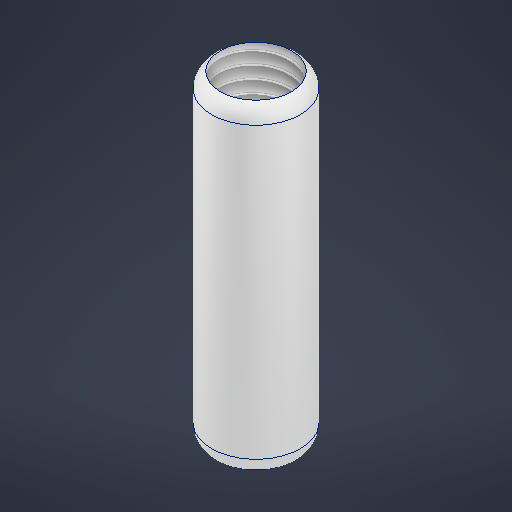
# Autodesk Inventor part: P_Gewindebuchse_M4_20
Saved by Autodesk Inventor 2026 (Build 300175000, 175)
## iProperties
Created: 2025-04-26
Part Number: P_Gewindebuchse_M4_20
Material: Aluminium 6061
Document SubType Name: Modeling
Designer: FAL
Density: 2.7 g/cm^3
Appearance: Aluminium - flach
Author: FAL
Autodesk Inventor part; units mm, degrees
ref_plane "YZ Plane" through (0, 0, 0) normal (1, 0, 0) x (0, 1, 0)
ref_plane "XZ Plane" through (0, 0, 0) normal (0, 1, 0) x (-1, 0, 0)
ref_plane "XY Plane" through (0, 0, 0) normal (0, 0, 1) x (1, 0, 0)
sketch "Skizze1" plane through (0, 0, 0) normal (0, 0, 1) x (1, 0, 0)
  circle A0 centre (0, 0) radius 2.5
  circle A1 centre (0, 0) radius 2
  dimension "d0" = 5
  dimension "d1" = 4
  constraints: 2 centre point, 2 coincident
  measures "d0" diameter of A0
  measures "d1" diameter of A1
extrude "Extrusion1" add sketch "Skizze1" along normal blind 18
thread "Gewinde1" size "M4x0.7" class "6H" standard "ANSI Metric M Profile" full length
fillet "Rundung1" radius 1 2 edges at (-2.5, 0, 18) (-2.5, 0, 0)
